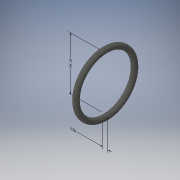
# Autodesk Inventor part: ORPP35-S
Saved by Autodesk Inventor 2019 (Build 230136000, 136)
## iProperties
Created: 2023-07-21
Part Number: ORPP35-S
Material: Generic
Catalog Web Link: www.cadenas.de
Description: ORPP ORGG-O-Rings
Vendor: TOHATSU
Document SubType Name: Modeling
Designer: psAdmin
Manufacturer: TOHATSU
Mass: 1.55874 g
Surface Area: 13.1957 cm^2
Volume: 1.15462 cm^3
Density: 1.35 g/cm^3
Appearance: PSOLRGB-94-94-91
Category: PARTsolutions
Company: TOHATSU
Title: ORPP35-S
Author: Cadenas PARTsolutions
Comments: O-Rings
PSOL_IDENT_0: {$CADENAS_DATA/23d-libs/tohatsu/spring_screw_washer/seal-materials/o-rings/orpp_orgg.prj},162 {VTYP=
PSOL_IDENT_1: 3D},{NB=ORPP35-S},{LINA=ORPP35-S},{NN=ORPP ORGG},{DATE=19.07.2023 02:54:23},{GEOMDATE=16.12.2022 07:
PSOL_IDENT_2: 08:00},{VERSION=},{LINEID=260},{WBVAR=MA},{WBNUMERIC=}  {NB=ORPP35-S},{LINA=ORPP35-S},{KT=DUMMY},{PN=
PSOL_IDENT_3: ORPP35-S},{TYPE=ORPP},{NO=35},{MA=S},{ROHS=NO},{QU=1350},{PS=活動用},{D=34.7},{T=3.5},{JISNO=P35},{WED=
PSOL_IDENT_4: 網站},{URL=https://www.tohatsu.com.tw}
NB: ORPP35-S
NN: ORPP ORGG
NT: O-Rings
NBSYN: $PN.
LINA: ORPP35-S
CATALOG: TOHATSU
PN: ORPP35-S
TYPE: ORPP
NO: 35
MA: SILICONE
ROHS: NO
PS: For events
WED: 網站
SUPPLIER: TOHATSU
ARTICLENO: ORPP35-S
BOMINFO: ORPP35-S
CREATOR: CADENAS GmbH
Autodesk Inventor part; units mm, degrees
ref_plane "YZ Plane" through (0, 0, 0) normal (1, 0, 0) x (0, 1, 0)
ref_plane "XZ Plane" through (0, 0, 0) normal (0, 1, 0) x (-1, 0, 0)
ref_plane "XY Plane" through (0, 0, 0) normal (0, 0, 1) x (1, 0, 0)
sketch "__1" plane through (0, 0, 0) normal (0, 0, 1) x (1, 0, 0)
  line L0 (35, 0) -> (-35, 0)
  circle A0 centre (1.75, 19.1) radius 1.75
  constraints: 2 end point, 1 centre point
revolve "Revolution1" add sketch "__1" angle 360 about axis through (35, 0, 0) along (1, 0, 0)
body "Solid1"
